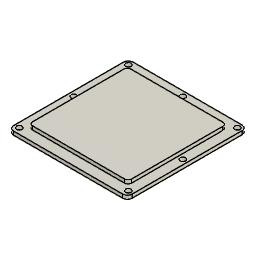
Rear Fan Mount - Blank (Autodesk Fusion 360 design; units mm, degrees)
Autodesk Fusion 360 part; units mm, degrees
sketch "Sketch1" plane through (0, 0, 0) normal (0, 0, 1) x (1, 0, 0) in component "Rear Fan Mount - 80mm"
  line L0 (-45.75, 45.75) -> (45.75, 45.75) construction
  line L1 (45.75, 45.75) -> (45.75, -45.75) construction
  line L2 (45.75, -45.75) -> (-45.75, -45.75) construction
  line L3 (-45.75, -45.75) -> (-45.75, 45.75) construction
  circle A0 centre (-45.75, 45.75) radius 4
  circle A1 centre (45.75, 45.75) radius 4
  circle A2 centre (-45.75, 0) radius 4
  circle A3 centre (0, 45.75) radius 4
  circle A4 centre (45.75, 0) radius 4
  circle A5 centre (-45.75, 45.75) radius 2.3
  circle A6 centre (0, 45.75) radius 2.3
  circle A7 centre (45.75, 45.75) radius 2.3
  circle A8 centre (-45.75, 0) radius 2.3
  circle A9 centre (45.75, 0) radius 2.3
  circle A10 centre (-45.75, -45.75) radius 2.3
  circle A11 centre (45.75, -45.75) radius 2.3
  line L4 (0, 70.061) -> (0, -70.061) construction
  line L5 (-88.2997, 0) -> (-84.09, 0)
  line L6 (-84.09, 0) -> (84.09, 0) construction
  line L7 (-45.75, -39.1372) -> (-45.75, -56.9142) construction
  line L8 (45.75, -34.6914) -> (45.75, -57.3902) construction
  circle A12 centre (-45.75, -46.5) radius 4
  circle A13 centre (45.75, -46.5) radius 4
  line L9 (49.75, -45.75) -> (49.75, -46.5)
  line L10 (-49.75, -45.75) -> (-49.75, -46.5)
  line L11 (-49.75, 49.75) -> (49.75, 49.75)
  line L12 (49.75, 49.75) -> (49.75, -50.5)
  line L13 (49.75, -50.5) -> (-49.75, -50.5)
  line L14 (-49.75, -50.5) -> (-49.75, 49.75)
  point P0 (0, -45.75)
  dimension "d1_1" = 8
  dimension "d2_1" = 8
  dimension "d5_1" = 8
  dimension "d6_1" = 8
  dimension "d7_1" = 8
  dimension "d8_1" = 4.6
  dimension "d9_1" = 4.6
  dimension "d10_1" = 4.6
  dimension "d11_1" = 4.6
  dimension "d12_1" = 4.6
  dimension "d13_1" = 4.6
  dimension "d14_1" = 4.6
  dimension "d42_1" = 91.5
  dimension "d43_1" = 91.5
  dimension "d48_1" = 8
  dimension "d49_1" = 8
  dimension "d55_1" = 91.5
  dimension "d56_1" = 45.75
  dimension "d58_1" = 45.75
  dimension "d59_1" = 100.25
  dimension "d4" = 4.75
  dimension "d16" = 45.75
  constraint horizontal L0
  constraint vertical L1
  constraint horizontal L2
  constraint vertical L3
  constraint coincident L0.start L3.end
  constraint coincident L0.end L1.start
  constraint midpoint L3 A2.centre
  constraint midpoint L0 A3.centre
  constraint midpoint L1 A4.centre
  constraint concentric A0 A5
  constraint concentric A3 A6
  constraint concentric A2 A8
  constraint concentric A4 A9
  constraint vertical L4
  constraint midpoint origin L4
  constraint parallel L0 L5
  constraint parallel L0 L6
  constraint midpoint origin L6
  constraint midpoint L2 P0
  constraint coincident L4 P0
  constraint coincident A4.centre L6
  constraint coincident L3 L7.start
  constraint perpendicular L2 L7
  constraint coincident L1 L8.start
  constraint parallel L1 L8
  constraint coincident L7 A12.centre
  constraint coincident L8 A13.centre
  constraint coincident A13 L9.end
  constraint tangent A13 L9
  constraint coincident A12 L10.end
  constraint tangent A12 L10
  constraint horizontal L11
  constraint vertical L12
  constraint horizontal L13
  constraint vertical L14
  constraint tangent A0 L11
  constraint tangent A0 L14
  constraint tangent A13 L12
  constraint tangent A12 L13
  constraint tangent A13 L13
  measures "d1_1" diameter of A0
  measures "d2_1" diameter of A1
  measures "d5_1" diameter of A2
  measures "d6_1" diameter of A3
  measures "d7_1" diameter of A4
  measures "d8_1" diameter of A5
  measures "d9_1" diameter of A6
  measures "d10_1" diameter of A7
  measures "d11_1" diameter of A8
  measures "d12_1" diameter of A9
  measures "d13_1" diameter of A10
  measures "d14_1" diameter of A11
  measures "d42_1" distance of L0.end L1.end
  measures "d43_1" distance of L0.start L0.end
  measures "d48_1" diameter of A12
  measures "d49_1" diameter of A13
  measures "d55_1" distance of L2.end L1.end
  measures "d56_1" distance of A4.centre L1.end
  measures "d58_1" distance of L1 L4
  measures "d59_1" distance of L11 L13
  measures "d4" distance of L2.end L13
  measures "d16" distance of L2.end A2.centre
extrude "Extrude5" add sketch "Sketch1" along normal blind 3 contours A0 | A2 | A4 | A3 | A0 A1 A12 A13 L9 L10 L11 L12 L13 L14 | A1 | A12 | A13 in component "Rear Fan Mount - 80mm"
sketch "Sketch1 (1)" plane through (0, 0, 3) normal (0, 0, 1) x (1, 0, 0) in component "Rear Fan Mount - 80mm"
  circle A0 centre (45.75, 45.75) radius 2.3
  circle A1 centre (-45.75, 45.75) radius 2.3
  circle A2 centre (-45.75, -45.75) radius 2.3
  circle A3 centre (45.75, -45.75) radius 2.3
  line L0 (0, 49.75) -> (0, -49.75) construction
  line L1 (-50.55, 0) -> (48.95, 0) construction
  line L2 (-40.3667, 40.75) -> (40.3667, 40.75)
  line L3 (-41.55, 40.75) -> (-41.55, -41.5)
  line L4 (41.55, -41.5) -> (41.55, 40.75)
  line L5 (-40.3667, 40.75) -> (40.3667, -39.9833) construction
  line L6 (-40.3667, -39.9833) -> (40.3667, 40.75) construction
  circle A4 centre (-35.75, 35.5) radius 2.3
  circle A5 centre (-35.75, -36) radius 2.3
  circle A6 centre (35.75, 35.5) radius 2.3
  circle A7 centre (35.75, -36) radius 2.3
  line L7 (-40.05, -0.25) -> (40.05, -0.25) construction
  circle A8 centre (0, -0.25) radius 38.5
  line L8 (41.55, 40.75) -> (-41.55, 40.75)
  circle A9 centre (45.75, -45.75) radius 4
  circle A10 centre (-45.75, -45.75) radius 4
  circle A11 centre (45.75, 45.75) radius 4
  circle A12 centre (-45.75, 45.75) radius 4
  circle A13 centre (45.75, 0) radius 2.3
  circle A14 centre (-45.75, 0) radius 2.3
  circle A15 centre (45.75, -45.75) radius 2.3
  circle A16 centre (45.75, 45.75) radius 2.3
  circle A17 centre (-45.75, -45.75) radius 2.3
  circle A18 centre (-45.75, 45.75) radius 2.3
  circle A19 centre (0, 45.75) radius 2.3
  line L9 (-49.75, 45.75) -> (-49.75, -46.5)
  arc A20 (-49.75, -46.5) -> (-45.75, -50.5) centre (-45.75, -46.5) ccw
  line L10 (-45.75, -50.5) -> (45.75, -50.5)
  arc A21 (45.75, -50.5) -> (49.75, -46.5) centre (45.75, -46.5) ccw
  line L11 (49.75, -46.5) -> (49.75, 45.75)
  arc A22 (49.75, 45.75) -> (45.75, 49.75) centre (45.75, 45.75) ccw
  line L12 (45.75, 49.75) -> (-45.75, 49.75)
  arc A23 (-45.75, 49.75) -> (-49.75, 45.75) centre (-45.75, 45.75) ccw
  line L13 (-41.55, -41.5) -> (-41.1784, -41.5)
  line L14 (0, 59.4728) -> (0, -59.4728) construction
  line L15 (-45.75, -45.75) -> (45.75, -45.75) construction
  line L16 (41.55, -41.5) -> (41.55, -41.75)
  line L17 (41.55, -41.75) -> (-41.55, -41.75)
  line L18 (-41.55, -41.75) -> (-41.55, -41.5)
  line L19 (41.55, 42.25) -> (41.55, 40.75)
  line L20 (41.55, 40.75) -> (-41.55, 40.75)
  line L21 (-41.55, 40.75) -> (-41.55, 42.25)
  point P0 (0, 40.75)
  point P1 (-30, 0)
  dimension "d28_1" = 4.6
  dimension "d29_1" = 4.6
  dimension "d30_1" = 4.6
  dimension "d31_1" = 4.6
  dimension "d32_1" = 71.5
  dimension "d33_1" = 71.5
  dimension "d39_1" = 77
  dimension "d131_1" = 4.2
  dimension "d132_1" = 82.9
  dimension "d134_1" = 4
  dimension "d139_1" = 9
  dimension "d140_1" = 80.7333
  dimension "d141_1" = 1.1833
  dimension "d142_1" = 1.1833
  dimension "d143_1" = 1.7667
  dimension "d144_1" = 1.1833
  dimension "d145_1" = 5.75
  dimension "d147_1" = 71.5
  constraint horizontal L2
  constraint midpoint L2 P0
  constraint coincident L0 P0
  constraint coincident L1 P1
  constraint perpendicular L1 L3
  constraint perpendicular L1 L4
  constraint symmetric L0 L3 L4
  constraint horizontal A4.centre A6.centre
  constraint vertical A4.centre A5.centre
  constraint vertical A6.centre A7.centre
  constraint horizontal A5.centre A7.centre
  constraint symmetric L0 A4.centre A6.centre
  constraint symmetric A6.centre A7.centre L7
  constraint coincident L7 A8.centre
  constraint coincident L0 A8.centre
  constraint perpendicular L0 L8
  constraint coincident L3.start L8.end
  constraint perpendicular L3 L13
  constraint collinear L2 L8
  constraint perpendicular L10 L14
  constraint midpoint origin L14
  constraint collinear L0 L14
  constraint coincident A2.centre A10.centre
  constraint coincident A3.centre A9.centre
  constraint vertical L16
  constraint horizontal L17
  constraint vertical L18
  constraint collinear L4 L16
  constraint collinear L3 L18
  constraint vertical L19
  constraint horizontal L20
  constraint vertical L21
  constraint collinear L2 L20
  constraint collinear L4 L19
  constraint collinear L3 L21
  measures "d28_1" diameter of A4
  measures "d29_1" diameter of A5
  measures "d30_1" diameter of A6
  measures "d31_1" diameter of A7
  measures "d32_1" distance of A6.centre A7.centre
  measures "d33_1" distance of A5.centre A7.centre
  measures "d39_1" diameter of A8
  measures "d131_1" distance of L3 A14.centre
  measures "d134_1" distance of L15 L17
  measures "d139_1" distance of L2 L12
  measures "d140_1" distance of L5.end L6.start
  measures "d141_1" distance of L2.start L3
  measures "d142_1" distance of L2.end L4
  measures "d143_1" distance of L5.end L17
  measures "d144_1" distance of L5.end L4
  measures "d145_1" distance of A5.centre L17
  measures "d147_1" distance of A4.centre A6.centre
extrude "Extrude12" add sketch "Sketch1 (1)" along normal blind 3 contours L2 L3 L4 L8 L16 L17 L18 L20 | A4 | A5 | A6 | A7 | A8 in component "Rear Fan Mount - 80mm"
fillet "Fillet6" radius 3 4 edges at (-41.55, -41.75, 4.5) (41.55, -41.75, 4.5) (41.55, 40.75, 4.5) (-41.55, 40.75, 4.5) in component "Rear Fan Mount - 80mm"
component "Rear Fan Mount - 80mm" placed x (1, 0, 0) y (0, 1, 0) z (0, 0, 1) at (0, 0, 0)
equation "d33_1 = d32_1"
equation "d48_1 = d3_1"
equation "d49_1 = d3_1"
equation "d3_1 = 8 mm"
